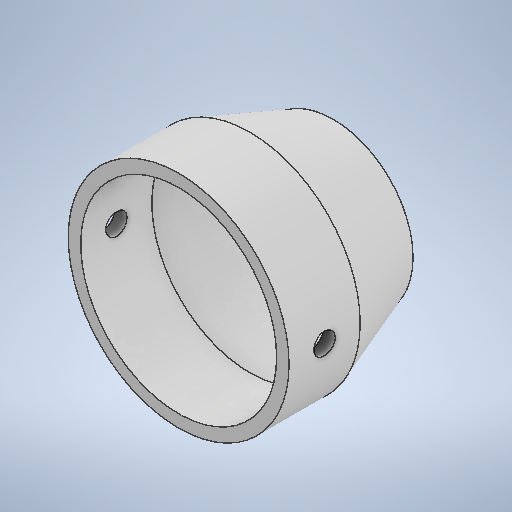
# Autodesk Inventor part: NOZZLE-ELIPTICO
Saved by Autodesk Inventor 2025.3 (Build 293356030, 356C)
## iProperties
Created: 2026-04-22
Part Number: NOZZLE-ELIPTICO
Material: Generic
Document SubType Name: Modeling
Designer: lstk1ng
Density: 1 g/cm^3
Appearance: Default
Author: lstk1ng
Autodesk Inventor part; units mm, degrees
ref_plane "YZ Plane" through (0, 0, 0) normal (1, 0, 0) x (0, 1, 0)
ref_plane "XZ Plane" through (0, 0, 0) normal (0, 1, 0) x (-1, 0, 0)
ref_plane "XY Plane" through (0, 0, 0) normal (0, 0, 1) x (1, 0, 0)
sketch "Sketch1" plane through (0, 0, 0) normal (0, 1, 0) x (-1, 0, 0)
  line L0 (-27.55, 40) -> (-27.55, 20)
  line L1 (-27.55, 20) -> (-20, 0)
  line L2 (0, 0) -> (0, 34.8486) construction
  line L3 (-20, 0) -> (0, 0)
  line L4 (0, -3.5) -> (-22.4198, -3.5)
  line L5 (-22.4198, -3.5) -> (-31.05, 20)
  line L6 (-31.05, 20) -> (-31.05, 40)
  line L7 (0, -3.5) -> (0, 0)
  line L8 (-27.55, 40) -> (-31.05, 40)
  dimension "d17" = 55.1
  dimension "d19" = 20
  dimension "d32" = 40
  dimension "d37" = 20
  constraints: 18 end point, 3 vertical, 2 horizontal
  measures "d17" diameter of L0 L2
  measures "d19" distance of L2.start L1.end
  measures "d32" distance from line of L3 L0.start
  measures "d37" distance of L5.end L6.end
revolve "Revolution1" add sketch "Sketch1" angle 360 about axis through (0, 0, 0) along (0, 0, 1)
sketch "Sketch5" plane through (0, 0, 0) normal (1, 0, 0) x (0, 1, 0)
  line L0 (27.55, 40) -> (-27.55, 40) projected
  line L1 (0, 40) -> (0, 30) construction
  circle A0 centre (0, 30) radius 3
  point P0 (0, 0)
  dimension "d27" = 10
  dimension "d28" = 6
  constraints: 2 end point, 1 centre point, 1 coincident, 1 midpoint, 1 vertical
  measures "d27" distance of L1.start L1.end
  measures "d28" diameter of A0
extrude "Extrusion4" cut sketch "Sketch5" along normal through all both and the other way through all
sketch "Sketch6" plane through (0, 0, -3.5) normal (0, 0, -1) x (-1, 0, 0)
  ellipse E0 centre (0, 0) end of major axis (-15, 0) minor radius 12.5
  dimension "d33" = 12.5
  dimension "d34" = 15
  constraints: 1 coincident, 2 other
extrude "Extrusion5" cut sketch "Sketch6" against normal blind 10
body "Solid1"
